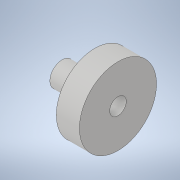
# Autodesk Inventor part: Flex_Bushing
Saved by Autodesk Inventor 2021 (Build 250183000, 183)
## iProperties
Created: 2020-10-19
Part Number: Flex_Bushing
Material: Generic
Document SubType Name: Modeling
Designer: PhotonUser
Density: 1 g/cm^3
Appearance: Default
Author: PhotonUser
Autodesk Inventor part; units mm, degrees
ref_plane "YZ Plane" through (0, 0, 0) normal (1, 0, 0) x (0, 1, 0)
ref_plane "XZ Plane" through (0, 0, 0) normal (0, 1, 0) x (-1, 0, 0)
ref_plane "XY Plane" through (0, 0, 0) normal (0, 0, 1) x (1, 0, 0)
sketch "Sketch1" plane through (0, 0, 0) normal (1, 0, 0) x (0, 1, 0)
  circle A0 centre (0, 0) radius 5.0038
  circle A1 centre (0, 0) radius 3.4036
  dimension "d0" = 10.0076
  dimension "d1" = 6.8072
  constraints: 2 centre point, 2 coincident
  measures "d0" diameter of A0
  measures "d1" diameter of A1
extrude "Extrusion1" add sketch "Sketch1" along normal blind 13.5128
sketch "Sketch2" plane through (13.5128, 0, 0) normal (1, 0, 0) x (0, 0, -1)
  circle A0 centre (0, 0) radius 15.875
  circle A1 centre (0, 0) radius 3.4036
  dimension "d4" = 31.75
  dimension "d7" = 6.8072
  constraints: 2 centre point, 2 coincident
  measures "d4" diameter of A0
  measures "d7" diameter of A1
extrude "Extrusion2" add sketch "Sketch2" along normal blind 9.525
body "Solid1"
